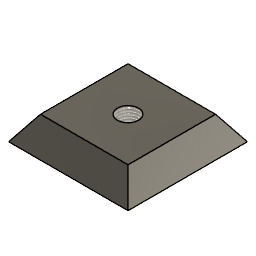
Base (Autodesk Fusion 360 design; units mm, degrees)
part number: 2026-02-13-11-14-04-177
Autodesk Fusion 360 part; units mm, degrees
sketch "Sketch1" plane through (0, 0, 0) normal (0, 0, 1) x (1, 0, 0)
  line L0 (75, 75) -> (-75, 75)
  line L1 (-75, 75) -> (-75, -75)
  line L2 (-75, -75) -> (75, -75)
  line L3 (75, -75) -> (75, 75)
  line L4 (75, 75) -> (-75, -75) construction
  line L5 (-75, 75) -> (75, -75) construction
  dimension "d3" = 150
  dimension "d4" = 150
  constraint horizontal L0
  constraint perpendicular L0 L1
  constraint parallel L0 L2
  constraint parallel L1 L3
  constraint coincident L4 origin
  constraint coincident L5 origin
  measures "d3" distance of L1.end L2.end
  measures "d4" distance of L0.end L1.end
ref_plane "WorkPlane1" through (0, 0, 30) normal (0, 0, 1) x (1, 0, 0)
sketch "Sketch2" plane through (0, 0, 30) normal (0, 0, 1) x (1, 0, 0)
  line L0 (55, 55) -> (-55, 55)
  line L1 (-55, 55) -> (-55, -55)
  line L2 (-55, -55) -> (55, -55)
  line L3 (55, -55) -> (55, 55)
  line L4 (55, 55) -> (-55, -55) construction
  line L5 (-55, 55) -> (55, -55) construction
  dimension "d10" = 110
  dimension "d11" = 110
  constraint horizontal L0
  constraint perpendicular L0 L1
  constraint parallel L0 L2
  constraint parallel L1 L3
  constraint coincident L4 origin
  constraint coincident L5 origin
  measures "d10" distance of L0.start L2.end
  measures "d11" distance of L1.end L2.end
loft "Loft1" add profiles "Sketch1", "Sketch2" section 1 section 2
ref_plane "WorkPlane2" through (0, 0, 30) normal (0, 0, 1) x (1, 0, 0)
sketch "Sketch4" plane through (0, 0, 30) normal (0, 0, 1) x (1, 0, 0)
  circle A0 centre (0, 0) radius 15
  dimension "d22" = 30
  constraint coincident A0.centre origin
  measures "d22" diameter of A0
extrude "Extrude3" cut sketch "Sketch4" against normal blind 20
thread "Thread2" "ISO Metric profile 30.0 M30x3.5 M30x3.5 6H" major diameter 30.3925 minor diameter 26.491 pitch 3.5 angle 60 resizes the face on face at (14.9814, -0.7477, 16.6667)
